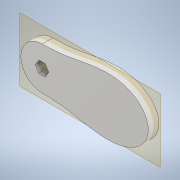
# Autodesk Inventor part: Disc Cam
Saved by Autodesk Inventor 2020.2 (Build 242310000, 310)
## iProperties
CustomPartVersion: 1
Created: 2020-01-13
Part Number: Disc Cam
Material: Stainless Steel, Austenitic
Document SubType Name: Modeling
Designer: robst
Manufacturer: Standard
Standards Organization: Custom
Density: 1 g/cm^3
Appearance: Steel
Author: robst
Autodesk Inventor part; units mm, degrees
ref_plane "YZ Plane" through (0, 0, 0) normal (1, 0, 0) x (0, 1, 0)
ref_plane "XZ Plane" through (0, 0, 0) normal (0, 1, 0) x (-1, 0, 0)
sketch "Main Sketch" plane through (0, 0, 0) normal (0, 0, 1) x (1, 0, 0)
  spline S0 degree 5 poles (0, 25.4) (2.1287, 25.4547) (7.6937, 25.5687) (25.2021, 26.4337) (31.4551, 28.162) (47.6615, 30.7176) (58.0563, 32.7726) (69.038, 34.1869) (78.7854, 34.6637) (88.084, 34.1038) (96.7063, 32.4528) (104.5913, 29.7259) (111.5026, 26.0227) (117.2575, 21.5254) (121.7221, 16.4677) (124.857, 11.0847) (126.6951, 5.5611) (127.2978, 0) (126.6951, -5.5611) (124.857, -11.0847) (121.722, -16.4677) (117.2576, -21.5254) (111.5024, -26.0226) (104.5919, -29.7259) (96.7046, -32.4526) (88.0883, -34.1042) (78.7741, -34.6626) (69.0685, -34.1898) (57.9701, -32.7645) (47.7056, -30.7009) (31.8315, -28.2651) (26.7281, -26.5857) (0.9075, -25.139) (-0.6141, -25.5787) (-4.7459, -25.0671) (-7.6748, -24.2891) (-10.3732, -23.2661) (-12.729, -22.0581) (-14.9733, -20.6052) (-17.0415, -18.9278) (-18.9282, -17.0425) (-20.6052, -14.9708) (-22.0575, -12.7349) (-23.2677, -10.3595) (-24.2232, -7.8706) (-24.9132, -5.2955) (-25.3302, -2.6623) (-25.4697, 0) (-25.3302, 2.6623) (-24.9131, 5.2955) (-24.2232, 7.8706) (-23.2676, 10.3595) (-22.0577, 12.7348) (-20.6048, 14.9708) (-18.9291, 17.0424) (-17.0393, 18.928) (-14.9785, 20.6047) (-12.7169, 22.0592) (-10.4011, 23.2637) (-7.879, 24.1938) (-5.6065, 24.8682) (-2.9673, 25.2646) (-1.9182, 25.346) (-0.8469, 25.3782) (0, 25.4) knots 0 0 0 0 0 0 0.034985 0.056949 0.083497 0.10838 0.131817 0.154181 0.175782 0.196779 0.217199 0.236988 0.256072 0.274418 0.292076 0.309193 0.326014 0.342834 0.359952 0.377609 0.395956 0.41504 0.434828 0.455248 0.476246 0.497846 0.52021 0.543647 0.568531 0.595079 0.619362 0.641097 0.659873 0.675226 0.686825 0.698424 0.710023 0.721622 0.733221 0.74482 0.756419 0.768018 0.779617 0.791217 0.802816 0.814415 0.826014 0.837613 0.849212 0.860811 0.87241 0.884009 0.895608 0.907207 0.918806 0.930406 0.942005 0.953604 0.965203 0.976802 0.986081 1 1 1 1 1 1
  point P0 (34.3511, 28.4773)
  point P1 (47.9087, 30.8624)
  point P2 (59.4553, 32.8129)
  point P3 (69.7636, 34.0431)
  point P4 (79.3599, 34.4006)
  point P5 (88.4593, 33.7633)
  point P6 (97.0267, 32.0479)
  point P7 (104.869, 29.2522)
  point P8 (111.7328, 25.4833)
  point P9 (117.3941, 20.9508)
  point P10 (121.7242, 15.9225)
  point P11 (124.7128, 10.6545)
  point P12 (126.4389, 5.3238)
  point P13 (127, 0)
  point P14 (126.4389, -5.3238)
  point P15 (124.7128, -10.6545)
  point P16 (121.7242, -15.9225)
  point P17 (117.3941, -20.9508)
  point P18 (111.7328, -25.4833)
  point P19 (104.869, -29.2522)
  point P20 (97.0267, -32.0479)
  point P21 (88.4593, -33.7633)
  point P22 (79.3599, -34.4006)
  point P23 (69.7636, -34.0431)
  point P24 (59.4553, -32.8129)
  point P25 (47.9087, -30.8624)
  point P26 (34.3511, -28.4773)
  point P27 (18.2006, -26.3139)
  point P28 (0, -25.4)
  point P29 (-2.655, -25.2609)
  point P30 (-5.281, -24.8449)
  point P31 (-7.849, -24.1568)
  point P32 (-10.3311, -23.2041)
  point P33 (-12.7, -21.997)
  point P34 (-14.9297, -20.549)
  point P35 (-16.9959, -18.8759)
  point P36 (-18.8759, -16.9959)
  point P37 (-20.549, -14.9297)
  point P38 (-21.997, -12.7)
  point P39 (-23.2041, -10.3311)
  point P40 (-24.1568, -7.849)
  point P41 (-24.8449, -5.281)
  point P42 (-25.2609, -2.655)
  point P43 (-25.4, 0)
  point P44 (-25.2609, 2.655)
  point P45 (-24.8449, 5.281)
  point P46 (-24.1568, 7.849)
  point P47 (-23.2041, 10.3311)
  point P48 (-21.997, 12.7)
  point P49 (-20.549, 14.9297)
  point P50 (-18.8759, 16.9959)
  point P51 (-16.9959, 18.8759)
  point P52 (-14.9297, 20.549)
  point P53 (-12.7, 21.997)
  point P54 (-10.3311, 23.2041)
  point P55 (-7.849, 24.1568)
  point P56 (-5.281, 24.8449)
  point P57 (-2.655, 25.2609)
  constraints: 60 other
extrude "Cam" add sketch "Main Sketch" along normal blind 12.7
sketch "Sketch2" plane through (0, 0, 12.7) normal (0, 0, 1) x (1, 0, 0)
  line L0 (7.9189, 0) -> (3.9595, -6.858)
  line L1 (3.9595, -6.858) -> (-3.9595, -6.858)
  line L2 (-3.9595, -6.858) -> (-7.9189, 0)
  line L3 (-7.9189, 0) -> (-3.9595, 6.858)
  line L4 (-3.9595, 6.858) -> (3.9595, 6.858)
  line L5 (3.9595, 6.858) -> (7.9189, 0)
  point P0 (0, 0)
  point P1 (0, 0)
  dimension "d4" = 13.716
  constraints: 12 end point, 1 coincident, 1 horizontal, 13 other
  measures "d4" distance between parallel lines of L1 L4
extrude "Extrusion2" cut sketch "Sketch2" against normal through all
ref_plane "Work Plane1" through (0, 0, 6.35) normal (0, 0, 1) x (1, 0, 0)
body "Solid1"
